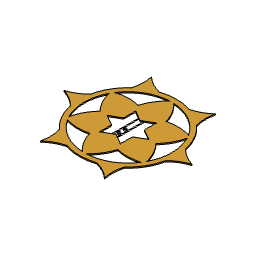
マリー_ヘイロー_mk1 v2 (Autodesk Fusion 360 design; units mm, degrees)
Autodesk Fusion 360 part; units mm, degrees
sketch "スケッチ1" plane through (0, 0, 0) normal (0, 0, 1) x (1, 0, 0)
  circle A0 centre (0, 0) radius 120 construction
  circle A1 centre (0, 0) radius 39 construction
  line L0 (0, 0) -> (120, 0) construction
  line L1 (0, 0) -> (26.25, 45.4663) construction
  line L2 (0, 0) -> (0, 22.5) construction
  line L3 (0, 22.5) -> (19.5, 33.775)
  line L4 (0, 0) -> (19.4856, 11.25) construction
  line L5 (19.4856, 11.25) -> (19.5, 33.775)
  line L6 (-19.4856, 11.25) -> (-19.5, 33.775)
  line L7 (0, 22.5) -> (-19.5, 33.775)
  line L8 (-19.4856, -11.25) -> (-39, 0)
  line L9 (-19.4856, 11.25) -> (-39, 0)
  line L10 (0, -22.5) -> (-19.5, -33.775)
  line L11 (-19.4856, -11.25) -> (-19.5, -33.775)
  line L12 (19.4856, -11.25) -> (19.5, -33.775)
  line L13 (0, -22.5) -> (19.5, -33.775)
  line L14 (19.4856, 11.25) -> (39, 0)
  line L15 (19.4856, -11.25) -> (39, 0)
  circle A2 centre (0, 0) radius 52.5 construction
  arc A3 (26.25, 45.4663) -> (3.8842, 81.908) centre (-53.2195, 21.7768) ccw
  arc A4 (-3.8842, 81.908) -> (-26.25, 45.4663) centre (53.2195, 21.7768) ccw
  arc A5 (-26.25, 45.4663) -> (-68.9922, 44.3178) centre (-45.469, -35.201) ccw
  arc A6 (-72.8765, 37.5901) -> (-52.5, 0) centre (7.7505, 56.9778) ccw
  arc A7 (-52.5, 0) -> (-72.8765, -37.5901) centre (7.7505, -56.9778) ccw
  arc A8 (-68.9922, -44.3178) -> (-26.25, -45.4663) centre (-45.469, 35.201) ccw
  arc A9 (-26.25, -45.4663) -> (-3.8842, -81.908) centre (53.2195, -21.7768) ccw
  arc A10 (3.8842, -81.908) -> (26.25, -45.4663) centre (-53.2195, -21.7768) ccw
  arc A11 (26.25, -45.4663) -> (68.9922, -44.3178) centre (45.469, 35.201) ccw
  arc A12 (72.8765, -37.5901) -> (52.5, 0) centre (-7.7505, -56.9778) ccw
  arc A13 (52.5, 0) -> (72.8765, 37.5901) centre (-7.7505, 56.9778) ccw
  arc A14 (68.9922, 44.3178) -> (26.25, 45.4663) centre (45.469, -35.201) ccw
  arc A15 (-3.8842, 81.908) -> (-68.9922, 44.3178) centre (0, 0) ccw
  arc A16 (-72.8765, 37.5901) -> (-72.8765, -37.5901) centre (0, 0) ccw
  arc A17 (-68.9922, -44.3178) -> (-3.8842, -81.908) centre (0, 0) ccw
  arc A18 (3.8842, -81.908) -> (68.9922, -44.3178) centre (0, 0) ccw
  arc A19 (72.8765, -37.5901) -> (72.8765, 37.5901) centre (0, 0) ccw
  arc A20 (68.9922, 44.3178) -> (3.8842, 81.908) centre (0, 0) ccw
  arc A21 (88.9993, 18.977) -> (120, 0) centre (140.7063, 68.6354) ccw
  arc A22 (120, 0) -> (88.9993, -18.977) centre (140.7063, -68.6354) ccw
  arc A23 (28.0651, 86.5641) -> (60, 103.923) centre (10.9132, 156.1729) ccw
  arc A24 (60, 103.923) -> (60.9342, 67.5871) centre (129.7931, 87.5375) ccw
  arc A25 (-60.9342, 67.5871) -> (-60, 103.923) centre (-129.7931, 87.5375) ccw
  arc A26 (-60, 103.923) -> (-28.0651, 86.5641) centre (-10.9132, 156.1729) ccw
  arc A27 (-88.9993, -18.977) -> (-120, 0) centre (-140.7063, -68.6354) ccw
  arc A28 (-120, 0) -> (-88.9993, 18.977) centre (-140.7063, 68.6354) ccw
  arc A29 (-28.0651, -86.5641) -> (-60, -103.923) centre (-10.9132, -156.1729) ccw
  arc A30 (-60, -103.923) -> (-60.9342, -67.5871) centre (-129.7931, -87.5375) ccw
  arc A31 (60.9342, -67.5871) -> (60, -103.923) centre (129.7931, -87.5375) ccw
  arc A32 (60, -103.923) -> (28.0651, -86.5641) centre (10.9132, -156.1729) ccw
  arc A33 (28.0651, 86.5641) -> (-28.0651, 86.5641) centre (0, 0) ccw
  arc A34 (88.9993, 18.977) -> (60.9342, 67.5871) centre (0, 0) ccw
  arc A35 (60.9342, -67.5871) -> (88.9993, -18.977) centre (0, 0) ccw
  arc A36 (-28.0651, -86.5641) -> (28.0651, -86.5641) centre (0, 0) ccw
  arc A37 (-60.9342, 67.5871) -> (-88.9993, 18.977) centre (0, 0) ccw
  arc A38 (-88.9993, -18.977) -> (-60.9342, -67.5871) centre (0, 0) ccw
  line L16 (-5, 25.391) -> (-5, -25.391)
  line L17 (5, 25.391) -> (5, -25.391)
  circle A39 centre (0, -17) radius 2.6
  circle A40 centre (0, -5) radius 2.6
  arc A41 (-5, 21.9374) -> (-5, -21.9374) centre (0, 0) ccw
  arc A42 (5, -21.9374) -> (5, 21.9374) centre (0, 0) ccw
  dimension "d2" = 240
  dimension "d3" = 182
  dimension "d4" = 164
  dimension "d5" = 78
  dimension "d6" = 45
  dimension "d7" = 60
  dimension "d9" = 360
  dimension "d10" = 105
  dimension "d12" = 360
  dimension "d14" = 360
  dimension "d17" = 10
  dimension "d18" = 5.2
  dimension "d19" = 5.2
  constraint coincident A0.centre A1.centre
  constraint concentric A0 A15
  constraint concentric A1 A15
  constraint coincident A0 L0.end
  constraint horizontal L0
  constraint coincident A1 L3.end
  constraint perpendicular L0 L2
  constraint symmetric L1 A0.centre A1.centre
  constraint symmetric L1 L2.end L4.end
  constraint concentric A2 A41
  constraint coincident A2 L1.end
  constraint coincident L3.end L1
  constraint symmetric L2 L1.end A4.end
  constraint symmetric L2 A3.end A4.start
  constraint symmetric L2 A3 A4
  constraint concentric A15 A16
  constraint concentric A16 A17
  constraint concentric A17 A18
  constraint concentric A18 A19
  constraint concentric A19 A20
  constraint coincident A21.start A37
  constraint symmetric A21.end L0 A22.start
  constraint symmetric L0 A21.start A22.end
  constraint symmetric L0 A21 A22
  constraint concentric A33 A37
  constraint concentric A34 A37
  constraint concentric A35 A37
  constraint concentric A36 A37
  constraint concentric A37 A38
  constraint parallel L2 L16
  constraint parallel L2 L17
  constraint symmetric L2 L16 L17
  constraint coincident L7 L16.start
  constraint coincident L3 L17.start
  constraint coincident L10 L16.end
  constraint coincident L13 L17.end
  constraint coincident L16 A41.start
  constraint coincident L17 A42.end
  constraint coincident L17 A42.start
  constraint concentric A41 A42
  constraint coincident L16 A41.end
  measures "d2" diameter of A0
  measures "d3" diameter of A37
  measures "d4" diameter of A15
  measures "d5" diameter of A1
  measures "d6" diameter of A41
  measures "d7" angle of L0 L1
  measures "d10" diameter of A2
  measures "d17" distance of L16 L17
  measures "d18" diameter of A39
  measures "d19" diameter of A40
extrude "押し出し2" add sketch "スケッチ1" along normal blind 2 contours A21 A22 A23 A24 A25 A26 A27 A28 A29 A30 A31 A32 A33 A34 A35 A36 A37 A38 makes body 1
extrude "押し出し3" add sketch "スケッチ1" along normal blind 2 separate body contours L3 L7 L10 L13 L16 L17 makes body 2
extrude "押し出し1" [suppressed]
equation "d4 = d3 - 18 mm"
